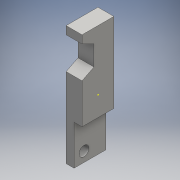
# Autodesk Inventor part: promo_hold2
Saved by Autodesk Inventor 2016 (Build 200138000, 138)
## iProperties
Created: 2016-05-12
Part Number: promo_hold2
Material: 一般
Document SubType Name: Modeling
Designer: 宏太
Density: 1 g/cm^3
Appearance: 既定
Mass: 0.612183 g
Surface Area: 7.01723 cm^2
Volume: 0.612183 cm^3
Author: 宏太
Autodesk Inventor part; units mm, degrees
ref_plane "YZ Plane" through (0, 0, 0) normal (1, 0, 0) x (0, 1, 0)
ref_plane "XZ Plane" through (0, 0, 0) normal (0, 1, 0) x (-1, 0, 0)
ref_plane "XY Plane" through (0, 0, 0) normal (0, 0, 1) x (1, 0, 0)
sketch "スケッチ1" plane through (0, 0, 0) normal (0, 1, 0) x (-1, 0, 0)
  line L0 (-2, 15) -> (2, 15)
  line L1 (2, 15) -> (2, -15)
  line L2 (2, -15) -> (-2, -15)
  line L3 (-2, -15) -> (-2, 15)
  line L4 (-2, 15) -> (2, -15) construction
  line L5 (2, 15) -> (-2, -15) construction
  point P0 (0, 0)
  dimension "d0" = 4
  dimension "d1" = 30
  constraints: 12 end point, 2 midpoint, 2 parallel, 1 horizontal, 1 perpendicular
  measures "d0" distance of L1.end L2.end
  measures "d1" distance of L0.end L1.end
extrude "押し出し1" add sketch "スケッチ1" along normal mid plane 8
sketch "スケッチ2" plane through (2, -4, -15) normal (1, 0, 0) x (0, 0, -1)
  line L0 (0, 0) -> (-30, 0) projected
  line L1 (-28, 0) -> (-26.5, 3)
  line L2 (-26.5, 3) -> (-21.5, 3)
  line L3 (-21.5, 3) -> (-20, 0)
  line L4 (-30, 0) -> (-30, 8) projected
  line L5 (-28, 0) -> (-20, 0)
  point P0 (-15, 4)
  dimension "d4" = 5
  dimension "d5" = 3
  dimension "d6" = 2
  dimension "d7" = 10
  dimension "d8" = 3.5
  constraints: 8 end point, 2 point on line, 1 collinear, 1 parallel
  measures "d4" distance of L1.end L2.end
  measures "d5" vertical distance of L1.start L1.end
  measures "d6" distance of L0.end L1.start
  measures "d7" distance of L0.end L3.end
  measures "d8" distance from line of L4 L1.end
extrude "押し出し2" cut sketch "スケッチ2" against normal blind 5
sketch "スケッチ6" plane through (2, -4, -15) normal (1, 0, 0) x (0, 0, -1)
  line L0 (0, 0) -> (-20, 0) projected
  line L1 (0, 0) -> (-10, 0)
  line L2 (-10, 0) -> (-10, 8)
  line L3 (-10, 8) -> (0, 8)
  line L4 (0, 8) -> (0, 0)
  point P0 (-15, 4)
  dimension "d22" = 10
  dimension "d23" = 8
  constraints: 8 end point, 2 parallel, 1 horizontal, 1 perpendicular
  measures "d22" distance of L2.end L3.end
  measures "d23" distance of L1.end L2.end
extrude "押し出し6" cut sketch "スケッチ6" against normal blind 2
sketch "スケッチ7" plane through (0, -4, -15) normal (1, 0, 0) x (0, 0, -1)
  circle A0 centre (-2.5, 2.5) radius 1.25
  line L0 (0, 8) -> (0, 0) projected
  point P0 (-15, 4)
  dimension "d26" = 2.5
  dimension "d27" = 2.5
  constraints: 1 centre point
  measures "d26" diameter of A0
  measures "d27" distance from line of L0 A0.centre
extrude "押し出し7" cut sketch "スケッチ7" against normal blind 2
sketch "スケッチ8" plane through (2, -4, 15) normal (1, 0, 0) x (0, 0, -1)
  point P0 (15, 4)
